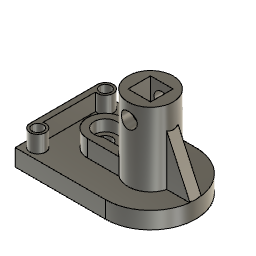
drawing_26 (Autodesk Fusion 360 design; units mm, degrees)
Autodesk Fusion 360 part; units mm, degrees
sketch "Sketch1" plane through (0, 0, 0) normal (0, 0, 1) x (1, 0, 0)
  line L0 (40, 40) -> (-40, 40)
  line L1 (-40, 40) -> (-40, -40)
  line L2 (-40, -40) -> (40, -40)
  line L3 (40, -40) -> (40, 40)
  line L4 (40, 40) -> (-40, -40) construction
  line L5 (-40, 40) -> (40, -40) construction
  dimension "d1" = 80
  dimension "d2" = 80
  constraint horizontal L0
  constraint perpendicular L0 L1
  constraint parallel L0 L2
  constraint parallel L1 L3
  constraint coincident L4 origin
  constraint coincident L5 origin
  measures "d1" distance of L1.end L2.end
  measures "d2" distance of L0.end L1.end
extrude "Extrude1" add sketch "Sketch1" along normal blind 15
sketch "Sketch2" plane through (0, 0, 15) normal (0, 0, 1) x (-1, 0, 0)
  line L0 (-40, 40) -> (-40, -40)
  line L1 (-40, -40) -> (40, -40)
  line L2 (40, -40) -> (40, 40)
  line L3 (40, 40) -> (-40, 40)
  circle A0 centre (-40, 0) radius 40
  dimension "d5" = 80
  measures "d5" diameter of A0
extrude "Extrude2" add sketch "Sketch2" against normal blind 15 contours L0 A0 picked at (-52.4116, 4.8712)
sketch "Sketch3" plane through (0, 0, 15) normal (0, 0, 1) x (-1, 0, 0)
  line L0 (-40, -40) -> (40, -40)
  line L1 (40, -40) -> (40, 40)
  line L2 (40, 40) -> (-40, 40)
  arc A0 (-40, 40) -> (-40, -40) centre (-40, 0) ccw
  circle A1 centre (-40, 0) radius 20
  dimension "d8" = 40
  constraint concentric A0 A1
  measures "d8" diameter of A1
extrude "Extrude3" add sketch "Sketch3" along normal blind 65 contours A1
sketch "Sketch4" plane through (0, 0, 80) normal (0, 0, 1) x (-1, 0, 0)
  circle A0 centre (-40, 0) radius 20
  line L0 (-50, -10) -> (-30, -10)
  line L1 (-30, -10) -> (-30, 10)
  line L2 (-30, 10) -> (-50, 10)
  line L3 (-50, 10) -> (-50, -10)
  line L4 (-50, -10) -> (-30, 10) construction
  line L5 (-30, -10) -> (-50, 10) construction
  point P0 (-40, 0)
  dimension "d11" = 20
  dimension "d12" = 20
  constraint horizontal L0
  constraint perpendicular L0 L1
  constraint parallel L0 L2
  constraint parallel L1 L3
  constraint coincident L4 P0
  constraint coincident L5 P0
  constraint coincident P0 A0.centre
  measures "d11" distance of L1.end L2.end
  measures "d12" distance of L0.end L1.end
extrude "Extrude4" cut sketch "Sketch4" against normal blind 155 contours L0 L1 L2 L3
ref_plane "WorkPlane1" through (40, -20, 56.6713) normal (0, -1, 0) x (-1, 0, 0)
sketch "Sketch5" plane through (40, -20, 56.6713) normal (0, -1, 0) x (1, 0, 0)
  line L0 (20, 23.3287) -> (-20, 23.3287)
  line L1 (-20, -41.6713) -> (20, -41.6713)
  line L2 (0, 23.3287) -> (0, 9.3287) construction
  circle A0 centre (0, 9.3287) radius 7
  dimension "d16" = 14
  dimension "d17" = 14
  constraint midpoint L0 L2.start
  constraint perpendicular L0 L2
  constraint coincident L2.end A0.centre
  measures "d16" distance of L2.start L2.end
  measures "d17" diameter of A0
extrude "Extrude9" cut sketch "Sketch5" against normal blind 110
extrude "Extrude5" cut sketch "Sketch5" against normal blind 60
sketch "Sketch6" plane through (0, 0, 15) normal (0, 0, 1) x (-1, 0, 0)
  circle A0 centre (-40, 0) radius 20
  line L0 (-40, -40) -> (40, -40)
  line L1 (40, -40) -> (40, 40)
  line L2 (40, 40) -> (-40, 40)
  arc A1 (-40, 40) -> (-40, -40) centre (-40, 0) ccw
  line L3 (-80, 0) -> (-55, 0) construction
  line L4 (-55, 0) -> (-55, -5) construction
  line L5 (-55, -5) -> (-55, 5) construction
  line L6 (-55, 5) -> (-79.6863, 5)
  line L7 (-55, 5) -> (-55, -5)
  line L8 (-79.6863, -5) -> (-55, -5)
  constraint midpoint A1 L3.start
  constraint horizontal L3
  constraint perpendicular L3 L4
  constraint perpendicular L3 L5
  constraint coincident A1 L6.end
  constraint perpendicular L5 L6
  constraint coincident A1 L8.start
  constraint perpendicular L7 L8
extrude "Extrude6" add sketch "Sketch6" along normal blind 45 contours A0 A1 L6 L8
sketch "Sketch7" plane through (0, -5, 0) normal (0, -1, 0) x (1, 0, 0)
  line L0 (59.3649, 15) -> (79.6863, 15)
  line L1 (79.6863, 15) -> (79.6863, 60)
  line L2 (79.6863, 60) -> (59.3649, 60)
  line L3 (59.3649, 60) -> (59.3649, 15)
  line L4 (79.6863, 15) -> (40, 15)
  line L5 (40, 15) -> (40, 0)
  line L6 (40, 0) -> (80, 0)
  line L7 (40, 0) -> (40, 15)
  line L8 (79.6863, 15) -> (40, 15)
  line L9 (79.6863, 15) -> (79.6863, 60)
  line L10 (80, 60) -> (79.6863, 60)
  line L11 (79.6863, 60) -> (79.6863, 15)
  line L12 (59.3649, 60) -> (80, 15)
  line L13 (79.6863, 15) -> (80, 15)
  line L14 (80, 15) -> (59.3649, 60)
  line L15 (80, 15) -> (80, 60)
  line L16 (59.3649, 60) -> (80, 60)
  constraint coincident L2.end L3.start
  constraint coincident L0.end L1.start
  constraint parallel L0 L13
  constraint coincident L10.start L15.end
  constraint perpendicular L10 L15
extrude "Extrude7" cut sketch "Sketch7" against normal blind 34 contours L1 L2 L9 L11 L12 L14 L16 | L1 L9 L10 L11 L12 L14 L15 L16
extrude "Extrude8" add 1 faces at (53.3333, 0, 80) along direction (0, 0, -1) blind 30
extrude "Extrude10" cut sketch "Sketch5" against normal blind 110
sketch "Sketch8" plane through (0, 0, 15) normal (0, 0, 1) x (-1, 0, 0)
  line L0 (-59.3649, -5) -> (-79.6863, -5)
  arc A0 (-79.6863, -5) -> (-40, -40) centre (-40, 0) ccw
  line L1 (-40, -40) -> (40, -40)
  line L2 (40, -40) -> (40, 40)
  line L3 (40, 40) -> (-40, 40)
  arc A1 (-40, 40) -> (-79.6863, 5) centre (-40, 0) ccw
  line L4 (-79.6863, 5) -> (-59.3649, 5)
  arc A2 (-59.3649, -5) -> (-59.3649, 5) centre (-40, 0) ccw
  line L5 (-30, -10) -> (-50, -10)
  line L6 (-50, -10) -> (-50, 10)
  line L7 (-50, 10) -> (-30, 10)
  line L8 (-30, 10) -> (-30, -10)
  circle A3 centre (-40, 0) radius 20
  line L9 (-40, 0) -> (0, 0) construction
  circle A4 centre (0, 0) radius 10
  circle A5 centre (0, 0) radius 6
  dimension "d30" = 40
  dimension "d31" = 20
  dimension "d32" = 12
  constraint coincident A0.centre A1.centre
  constraint perpendicular L8 L9
  constraint coincident L9.end A4.centre
  measures "d30" distance of A0.centre L9.end
  measures "d31" diameter of A4
  measures "d32" diameter of A5
extrude "Extrude11" cut sketch "Sketch8" against normal blind 45 contours A5
sketch "Sketch9" plane through (0, 0, 15) normal (0, 0, 1) x (-1, 0, 0)
  circle A0 centre (0, 0) radius 6
  line L0 (-59.3649, -5) -> (-79.6863, -5)
  arc A1 (-79.6863, -5) -> (-40, -40) centre (-40, 0) ccw
  line L1 (-40, -40) -> (40, -40)
  line L2 (40, -40) -> (40, 40)
  line L3 (40, 40) -> (-40, 40)
  arc A2 (-40, 40) -> (-79.6863, 5) centre (-40, 0) ccw
  line L4 (-79.6863, 5) -> (-59.3649, 5)
  arc A3 (-59.3649, -5) -> (-59.3649, 5) centre (-40, 0) ccw
  line L5 (-30, -10) -> (-50, -10)
  line L6 (-50, -10) -> (-50, 10)
  line L7 (-50, 10) -> (-30, 10)
  line L8 (-30, 10) -> (-30, -10)
  circle A4 centre (-40, 0) radius 20
  line L9 (0, -16) -> (-28, -16)
  line L10 (0, 16) -> (-28, 16)
  arc A5 (0, -16) -> (0, 16) centre (0, 0) ccw
  dimension "d35" = 32
  constraint coincident A0.centre A5.centre
  constraint horizontal L9
  constraint coincident A4 L9.end
  constraint coincident A3 L9.end
  constraint horizontal L10
  constraint coincident A4 L10.end
  measures "d35" diameter of A5
extrude "Extrude12" add sketch "Sketch9" along normal blind 15 contours A3 A4 L9 L10 A5
sketch "Sketch10" plane through (0, 0, 30) normal (0, 0, 1) x (-1, 0, 0)
  circle A0 centre (0, 0) radius 6
  line L0 (-28, -16) -> (0, -16)
  arc A1 (0, -16) -> (0, 16) centre (0, 0) ccw
  line L1 (0, 16) -> (-28, 16)
  arc A2 (-28, -16) -> (-28, 16) centre (-40, 0) ccw
  line L2 (-30, -10) -> (-50, -10)
  line L3 (-50, -10) -> (-50, 10)
  line L4 (-50, 10) -> (-30, 10)
  line L5 (-30, 10) -> (-30, -10)
  circle A3 centre (-40, 0) radius 20
  line L6 (0, 0) -> (-40, 0) construction
  line L7 (-40, 0) -> (-40, -8) construction
  line L8 (-40, 0) -> (-40, 8) construction
  circle A4 centre (-40, 0) radius 20
  line L9 (-40, 8) -> (-30, 8)
  line L10 (-21.6697, 8) -> (-6, 8)
  line L11 (-40, -8) -> (-30, -8)
  line L12 (-21.6697, -8) -> (-6, -8)
  arc A5 (-6, -8) -> (-6, 8) centre (0, 0) ccw
  dimension "d39" = 20
  dimension "d40" = 8
  dimension "d41" = 8
  constraint coincident A0.centre A1.centre
  constraint coincident A2.centre A3.centre
  constraint perpendicular L6 L7
  constraint perpendicular L7 L11
  constraint perpendicular L6 L8
  constraint perpendicular L8 L9
  constraint concentric A3 A4
  constraint coincident L5 L9.end
  constraint coincident A2 L10.start
  constraint collinear L9 L10
  constraint coincident L5 L11.end
  constraint coincident A2 L12.start
  constraint collinear L11 L12
  measures "d39" diameter of A5
  measures "d40" distance of A2.centre L7.end
  measures "d41" distance of A2.centre L8.end
extrude "Extrude13" cut sketch "Sketch10" against normal blind 10 contours A2 A3 A4 L10 L12 A5
sketch "Sketch11" plane through (0, 0, 15) normal (0, 0, 1) x (-1, 0, 0)
  line L0 (-28, 16) -> (0, 16)
  arc A0 (0, -16) -> (0, 16) centre (0, 0) ccw
  line L1 (0, -16) -> (-28, -16)
  arc A1 (-59.3649, -5) -> (-28, -16) centre (-40, 0) ccw
  line L2 (-59.3649, -5) -> (-79.6863, -5)
  arc A2 (-79.6863, -5) -> (-40, -40) centre (-40, 0) ccw
  line L3 (-40, -40) -> (40, -40)
  line L4 (40, -40) -> (40, 40)
  line L5 (40, 40) -> (-40, 40)
  arc A3 (-40, 40) -> (-79.6863, 5) centre (-40, 0) ccw
  line L6 (-79.6863, 5) -> (-59.3649, 5)
  arc A4 (-28, 16) -> (-59.3649, 5) centre (-40, 0) ccw
  line L7 (0, 0) -> (30, 0) construction
  line L8 (40, -40) -> (30, -40) construction
  line L9 (40, -40) -> (40, -30) construction
  line L10 (40, 40) -> (40, 30) construction
  line L11 (40, 40) -> (30, 40) construction
  line L12 (37, -30) -> (37, 30)
  line L13 (37, -19.6755) -> (32, -19.6755) construction
  line L14 (32, -23.2918) -> (32, 23.2918)
  arc A5 (37, 30) -> (32, 23.2918) centre (30, 30) ccw
  arc A6 (32, -23.2918) -> (37, -30) centre (30, -30) ccw
  dimension "d44" = 30
  dimension "d45" = 10
  dimension "d47" = 10
  dimension "d48" = 10
  dimension "d49" = 14
  dimension "d50" = 14
  dimension "d51" = 5
  constraint coincident A0.centre L7.start
  constraint horizontal L7
  constraint coincident L3.end L4.start
  constraint perpendicular L4 L8
  constraint perpendicular L3 L9
  constraint coincident L4.end L5.start
  constraint perpendicular L5 L10
  constraint perpendicular L10 L11
  constraint tangent L12 A5
  constraint vertical L12
  constraint coincident L12 L13.start
  constraint perpendicular L12 L13
  constraint perpendicular L13 L14
  measures "d44" distance of A0.centre L7.end
  measures "d45" distance of L3.end L8.end
  measures "d47" distance of L4.end L10.end
  measures "d48" distance of L4.end L11.end
  measures "d49" diameter of A6
  measures "d50" diameter of A5
  measures "d51" distance of L13.start L13.end
extrude "Extrude14" add sketch "Sketch11" along normal blind 15 contours L12 L14 A5 A6
sketch "Sketch12" plane through (0, 0, 30) normal (0, 0, 1) x (-1, 0, 0)
  arc A0 (32, -23.2918) -> (37, -30) centre (30, -30) ccw
  line L0 (37, -30) -> (37, 30)
  arc A1 (37, 30) -> (32, 23.2918) centre (30, 30) ccw
  line L1 (32, 23.2918) -> (32, -23.2918)
  circle A2 centre (30, -30) radius 5
  circle A3 centre (30, 30) radius 5
  dimension "d54" = 10
  dimension "d55" = 10
  constraint concentric A0 A2
  constraint concentric A1 A3
  measures "d54" diameter of A2
  measures "d55" diameter of A3
extrude "Extrude15" cut sketch "Sketch12" against normal blind 70 contours A2 | A3
sketch "Sketch13" plane through (0, 0, 0) normal (0, 0, -1) x (1, 0, 0)
  circle A0 centre (-30, 30) radius 5
  circle A1 centre (-30, -30) radius 5
  circle A2 centre (0, 0) radius 6
  line L0 (50, -10) -> (30, -10)
  line L1 (30, -10) -> (30, 10)
  line L2 (30, 10) -> (50, 10)
  line L3 (50, 10) -> (50, -10)
  line L4 (40, 40) -> (-40, 40)
  line L5 (-40, 40) -> (-40, -40)
  line L6 (-40, -40) -> (40, -40)
  arc A3 (40, -40) -> (40, 40) centre (40, 0) ccw
  circle A4 centre (40, 0) radius 14
  dimension "d58" = 28
  constraint concentric A3 A4
  measures "d58" diameter of A4
extrude "Extrude16" cut sketch "Sketch13" against normal blind 20 contours L0 A4 | L0 L1 L2 L3 A4 | L3 A4 | L1 A4 | L2 A4
equation "d9 = 80 mm - 15 mm"
equation "d20 = 60 mm - 15 mm"
